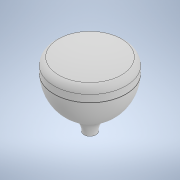
# Autodesk Inventor part: Рукоятка
Saved by Autodesk Inventor 2021 (Build 250183000, 183)
## iProperties
Created: 2021-04-19
Part Number: Рукоятка
Material: Типовые
Document SubType Name: Modeling
Designer: Данил
Density: 1 g/cm^3
Appearance: По умолчанию
Author: Данил
Autodesk Inventor part; units mm, degrees
ref_plane "YZ Plane" through (0, 0, 0) normal (1, 0, 0) x (0, 1, 0)
ref_plane "XZ Plane" through (0, 0, 0) normal (0, 1, 0) x (-1, 0, 0)
ref_plane "XY Plane" through (0, 0, 0) normal (0, 0, 1) x (1, 0, 0)
sketch "Эскиз1" plane through (0, 0, 0) normal (0, 0, 1) x (1, 0, 0)
  line L0 (0, 45) -> (0, -45)
  arc A0 (45, 32.9423) -> (0, 45) centre (0, -45) ccw
  line L1 (45, 32.9423) -> (45, 17.9423)
  arc A1 (20.0138, -23.3414) -> (45, 17.9423) centre (-4.9586, 19.9758) ccw
  arc A2 (20.0138, -23.3414) -> (7.5, -45) centre (32.5, -45) ccw
  line L2 (0, -45) -> (7.5, -45)
  point P0 (0, 0)
  point P1 (0, 0)
  dimension "d0" = 90
  dimension "d1" = 90
  dimension "d2" = 15
  dimension "d3" = 15
  dimension "d4" = 50
  dimension "d5" = 25
  constraints: 6 end point, 6 point on circle, 3 centre point, 2 coincident, 2 horizontal alignment, 2 line through centre, 2 vertical, 1 horizontal, 1 midpoint, 1 tangent
  measures "d0" distance of L0.start L0.end
  measures "d1" diameter of L1 L0
  measures "d2" distance of L1.start L1.end
  measures "d3" diameter of L2.end L0
  measures "d4" radius of A1
  measures "d5" radius of A2
revolve "Вращение1" add sketch "Эскиз1" angle 360 about axis through (0, 45, 0) along (0, -1, 0)
fillet "Сопряжение1" radius 10 2 edges at (-45, 32.9423, 0) (-45, 17.9423, 0)
sketch "Эскиз2" plane through (0, -45, 0) normal (0, -1, 0) x (1, 0, 0)
  circle A0 centre (0, 0) radius 7.5 projected
  point P0 (0, 0)
  constraints: 1 coincident
hole "Отверстие1" at (0, -45, 0) direction (0, 1, 0) diameter 8.9175 depth 21 tip angle 120 thread size "M10x1" class "6H" standard "ISO Metric profile"
